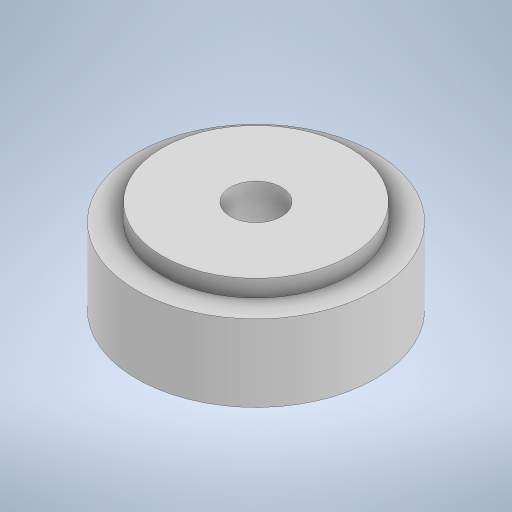
# Autodesk Inventor part: 6_Piston
Saved by Autodesk Inventor 2024.3 (Build 283343000, 343)
## iProperties
Created: 2024-04-26
Part Number: 6_Piston
Material: Genérico
Document SubType Name: Modeling
Designer: Cosmic Dinodog
Density: 1 g/cm^3
Appearance: Valor por defecto
Author: Cosmic Dinodog
Autodesk Inventor part; units mm, degrees
ref_plane "YZ Plane" through (0, 0, 0) normal (1, 0, 0) x (0, 1, 0)
ref_plane "XZ Plane" through (0, 0, 0) normal (0, 1, 0) x (-1, 0, 0)
ref_plane "XY Plane" through (0, 0, 0) normal (0, 0, 1) x (1, 0, 0)
sketch "Boceto1" plane through (0, 0, 0) normal (0, 0, 1) x (1, 0, 0)
  line L0 (0, 0) -> (9, 0) construction
  line L1 (9, 0) -> (9, 33)
  line L2 (42, 0) -> (42, 27)
  line L3 (42, 27) -> (33, 27)
  line L4 (33, 27) -> (33, 33)
  line L5 (33, 33) -> (9, 33)
  line L6 (42, 0) -> (42, 3) construction
  line L7 (42, 3) -> (40, 3) construction
  line L8 (40, 3) -> (37, 0)
  line L9 (40, 3) -> (43.5355, 3) construction
  line L10 (40, 3) -> (40, 0)
  line L11 (9, 0) -> (37, 0)
  line L12 (40, 0) -> (42, 0)
  line L13 (0, 0) -> (0, 41.2707) construction
  dimension "d0" = 9
  dimension "d1" = 33
  dimension "d2" = 33
  dimension "d3" = 27
  dimension "d4" = 9
  dimension "d5" = 3
  dimension "d6" = 2
  dimension "d7" = 135
  dimension "d8" = 6
  constraints: 28 end point, 5 horizontal, 5 perpendicular, 3 vertical, 1 point on line
  measures "d0" distance of L0.start L0.end
  measures "d1" distance of L0.end L2.start
  measures "d2" distance of L0.end L1.end
  measures "d3" distance of L2.start L2.end
  measures "d4" distance of L2.end L3.end
  measures "d5" distance of L2.start L6.end
  measures "d6" distance of L6.end L7.end
  measures "d7" angle of L8 L9
  measures "d8" distance of L3.end L4.end
revolve "Revolución1" add sketch "Boceto1" angle 360 about axis through (0, 0, 0) along (0, 1, 0)
